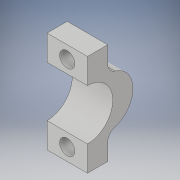
# Autodesk Inventor part: Klemme
Saved by Autodesk Inventor 2018.3 (Build 223284000, 284)
## iProperties
Created: 2018-11-22
Part Number: Klemme
Material: Generisch
Document SubType Name: Modeling
Designer: pgmadmin
Density: 1 g/cm^3
Appearance: Vorgabe
Author: pgmadmin
Autodesk Inventor part; units mm, degrees
ref_plane "YZ Plane" through (0, 0, 0) normal (1, 0, 0) x (0, 1, 0)
ref_plane "XZ Plane" through (0, 0, 0) normal (0, 1, 0) x (-1, 0, 0)
ref_plane "XY Plane" through (0, 0, 0) normal (0, 0, 1) x (1, 0, 0)
sketch "Skizze1" plane through (0, 0, 0) normal (1, 0, 0) x (0, 1, 0)
  line L0 (3.0012, 15.2548) -> (7.0012, 15.2548)
  line L1 (7.0012, -4.7452) -> (3.0012, -4.7452)
  arc A0 (3.0012, 0.2548) -> (3.0012, 10.2548) centre (3.0012, 5.2548) ccw
  arc A1 (7.0012, 0.2548) -> (7.0012, 10.2548) centre (7.0012, 5.2548) ccw
  line L2 (3.0012, -4.7452) -> (3.0012, 0.2548)
  line L3 (3.0012, 10.2548) -> (3.0012, 15.2548)
  line L4 (7.0012, 15.2548) -> (7.0012, 10.2548)
  line L5 (7.0012, 0.2548) -> (7.0012, -4.7452)
  point P0 (0, 0)
  dimension "d0" = 4
  dimension "d1" = 20
  dimension "d3" = 10
  constraints: 12 end point, 6 perpendicular, 4 point on circle, 2 centre point, 1 horizontal
  measures "d0" distance of L0.start L0.end
  measures "d1" distance between parallel lines of L1 L0
  measures "d3" diameter of A0
extrude "Extrusion1" add sketch "Skizze1" along normal blind 8
sketch "Skizze2" plane through (0, 7.0012, 15.2548) normal (0, 1, 0) x (1, 0, 0)
  line L0 (0, 0) -> (8, 0) projected
  line L1 (0, 20) -> (8, 20) projected
  line L2 (8, 20) -> (8, 15) projected
  line L3 (8, 5) -> (8, 0) projected
  point P0 (0, 15.2548)
  point P1 (4, 2.5)
  point P2 (4, 17.5)
  point P3 (4, 2.5)
  dimension "d6" = 2.5
  dimension "d7" = 2.5
  dimension "d8" = 4
  dimension "d9" = 4
  constraints: 1 coincident
  measures "d6" distance from line of L0 point (4, 2.5)
  measures "d7" distance from line of L1 point (4, 17.5)
  measures "d8" distance from line of L2 point (4, 17.5)
  measures "d9" distance from line of L3 point (4, 2.5)
hole "Bohrung1" at (4, 7.0012, 12.7548) at (4, 7.0012, -2.2452) direction (0, -1, 0) diameter 3 depth 8 tip angle 118
fillet "Rundung1" radius 2 2 edges at (4, 7.0012, 10.2548) (4, 7.0012, 0.2548)
